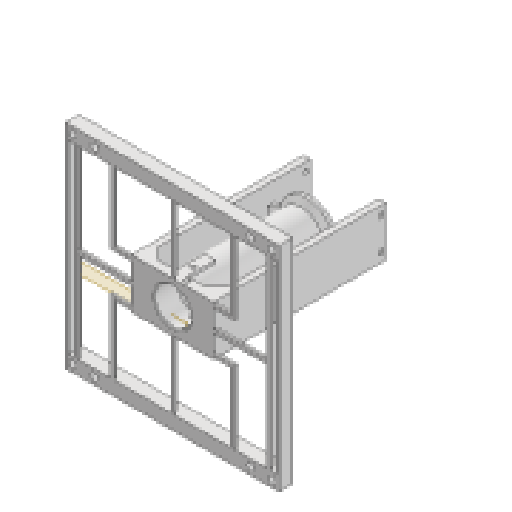
# Autodesk Inventor part: Flexible_tube_bolster_fixed_v3
Saved by Autodesk Inventor 2023 (Build 270158000, 158)
## iProperties
Created: 2021-01-08
Part Number: Flexible_tube_bolster_fixed_v3
Material: Generic
Document SubType Name: Modeling
Designer: CDT
Density: 1 g/cm^3
Appearance: Default
Author: CDT
Autodesk Inventor part; units mm, degrees
ref_plane "YZ Plane" through (0, 0, 0) normal (1, 0, 0) x (0, 1, 0)
ref_plane "XZ Plane" through (0, 0, 0) normal (0, 1, 0) x (-1, 0, 0)
ref_plane "XY Plane" through (0, 0, 0) normal (0, 0, 1) x (1, 0, 0)
ref_plane "Work Plane1" through (0, 0, 0) normal (0, 0, 1) x (1, 0, 0)
sketch "Sketch1" plane through (0, 0, 0) normal (0, 0, 1) x (1, 0, 0)
  line L0 (-30.0874, -48.0547) -> (89.9126, -48.0547)
  line L1 (89.9126, -48.0547) -> (89.9126, 71.9453)
  line L2 (89.9126, 71.9453) -> (-30.0874, 71.9453)
  line L3 (-30.0874, 71.9453) -> (-30.0874, -48.0547)
  circle A0 centre (-26.0874, 67.9453) radius 2
  circle A1 centre (85.9126, 67.9453) radius 2
  circle A2 centre (85.9126, -44.0547) radius 2
  circle A3 centre (-26.0874, -44.0547) radius 2
  circle A4 centre (-14.0874, 67.9453) radius 2
  circle A5 centre (73.9126, 67.9453) radius 2
  circle A6 centre (-14.0874, -44.0547) radius 2
  circle A7 centre (73.9126, -44.0547) radius 2
  point P0 (0, 0)
  dimension "d0" = 120
  dimension "d1" = 120
  dimension "d2" = 4
  dimension "d3" = 4
  dimension "d4" = 4
  dimension "d5" = 4
  dimension "d107" = 4
  dimension "d108" = 4
  dimension "d109" = 4
  dimension "d110" = 4
  dimension "d111" = 4
  dimension "d112" = 4
  dimension "d113" = 4
  dimension "d114" = 4
  dimension "d172" = 4
  dimension "d173" = 4
  dimension "d174" = 4
  dimension "d175" = 4
  dimension "d176" = 16
  dimension "d177" = 4
  dimension "d178" = 4
  dimension "d179" = 16
  dimension "d180" = 16
  dimension "d181" = 4
  dimension "d182" = 4
  dimension "d183" = 16
  constraints: 8 centre point, 8 end point, 2 parallel, 1 horizontal, 1 perpendicular
  measures "d0" distance of L2.end L0.start
  measures "d1" distance of L1.end L2.end
  measures "d2" diameter of A0
  measures "d3" diameter of A1
  measures "d4" diameter of A2
  measures "d5" diameter of A3
  measures "d107" distance from line of L1 A1.centre
  measures "d108" distance from line of L3 A0.centre
  measures "d109" distance from line of L3 A3.centre
  measures "d110" distance from line of L1 A2.centre
  measures "d111" distance from line of L2 A0.centre
  measures "d112" distance from line of L2 A1.centre
  measures "d113" distance from line of L0 A2.centre
  measures "d114" distance from line of L0 A3.centre
  measures "d172" diameter of A4
  measures "d173" diameter of A5
  measures "d174" diameter of A6
  measures "d175" diameter of A7
  measures "d176" distance from line of A6.centre L3
  measures "d177" distance from line of L0 A6.centre
  measures "d178" distance from line of L0 A7.centre
  measures "d179" distance from line of L1 A7.centre
  measures "d180" distance from line of L1 A5.centre
  measures "d181" distance from line of L2 A5.centre
  measures "d182" distance from line of L2 A4.centre
  measures "d183" distance from line of L3 A4.centre
extrude "Extrusion1" add sketch "Sketch1" along normal blind 5
sketch "Sketch2" plane through (0, 0, 5) normal (0, 0, 1) x (1, 0, 0)
  line L0 (-23.0874, -40.0547) -> (6.9126, -40.0547)
  line L1 (6.9126, -40.0547) -> (6.9126, 10.6953)
  line L2 (6.9126, 10.6953) -> (-23.0874, 10.6953)
  line L3 (-23.0874, 10.6953) -> (-23.0874, -40.0547)
  line L4 (89.9126, -48.0547) -> (89.9126, 71.9453) projected
  line L5 (-30.0874, 71.9453) -> (-30.0874, -48.0547) projected
  line L6 (-30.0874, -48.0547) -> (89.9126, -48.0547) projected
  line L7 (89.9126, 71.9453) -> (-30.0874, 71.9453) projected
  line L8 (-23.0874, 13.1953) -> (6.9126, 13.1953)
  line L9 (6.9126, 13.1953) -> (6.9126, 63.9453)
  line L10 (6.9126, 63.9453) -> (-23.0874, 63.9453)
  line L11 (-23.0874, 63.9453) -> (-23.0874, 13.1953)
  line L12 (82.9126, -40.0547) -> (52.9126, -40.0547)
  line L13 (52.9126, -40.0547) -> (52.9126, 10.6953)
  line L14 (52.9126, 10.6953) -> (82.9126, 10.6953)
  line L15 (82.9126, 10.6953) -> (82.9126, -40.0547)
  line L16 (82.9126, 13.1953) -> (52.9126, 13.1953)
  line L17 (52.9126, 13.1953) -> (52.9126, 63.9453)
  line L18 (52.9126, 63.9453) -> (82.9126, 63.9453)
  line L19 (82.9126, 63.9453) -> (82.9126, 13.1953)
  line L20 (-23.0874, -40.0547) -> (82.9126, -40.0547)
  line L21 (82.9126, -40.0547) -> (82.9126, -2.0547)
  line L22 (82.9126, -2.0547) -> (-23.0874, -2.0547)
  line L23 (-23.0874, -2.0547) -> (-23.0874, -40.0547)
  line L24 (-23.0874, 63.9453) -> (82.9126, 63.9453)
  line L25 (82.9126, 63.9453) -> (82.9126, 25.9453)
  line L26 (82.9126, 25.9453) -> (-23.0874, 25.9453)
  line L27 (-23.0874, 25.9453) -> (-23.0874, 63.9453)
  line L28 (82.9126, 11.9453) -> (52.9126, 11.9453)
  line L29 (52.9126, 11.9453) -> (52.9126, 11.9453)
  line L30 (52.9126, 11.9453) -> (82.9126, 11.9453)
  line L31 (82.9126, 11.9453) -> (82.9126, 11.9453)
  line L32 (11.9126, 11.9453) -> (-23.0874, 11.9453)
  line L33 (-23.0874, 11.9453) -> (-23.0874, 11.9453)
  line L34 (-23.0874, 11.9453) -> (11.9126, 11.9453)
  line L35 (11.9126, 11.9453) -> (11.9126, 11.9453)
  line L36 (-25.5874, -40.0547) -> (-30.0874, -40.0547)
  line L37 (-30.0874, -40.0547) -> (-30.0874, 63.9453)
  line L38 (-30.0874, 63.9453) -> (-25.5874, 63.9453)
  line L39 (-25.5874, 63.9453) -> (-25.5874, -40.0547)
  line L40 (89.9126, 63.9453) -> (85.4126, 63.9453)
  line L41 (85.4126, 63.9453) -> (85.4126, -40.0547)
  line L42 (85.4126, -40.0547) -> (89.9126, -40.0547)
  line L43 (89.9126, -40.0547) -> (89.9126, 63.9453)
  line L44 (-30.0874, -48.0547) -> (-44.0088, -48.0547)
  line L45 (-44.0088, -48.0547) -> (-44.0088, 71.9453)
  line L46 (-44.0088, 71.9453) -> (-30.0874, 71.9453)
  line L47 (-30.0874, 71.9453) -> (-30.0874, -48.0547)
  point P0 (0, 0)
  point P1 (6.9126, 63.9453)
  point P2 (6.9126, 25.9453)
  point P3 (52.9126, 25.9453)
  point P4 (52.9126, -2.0547)
  point P5 (6.9126, -2.0547)
  point P6 (-30.0874, 63.9453)
  point P7 (-30.0874, -40.0547)
  point P8 (89.9126, -40.0547)
  dimension "d9" = 7
  dimension "d10" = 8
  dimension "d13" = 8
  dimension "d15" = 7
  dimension "d19" = 7
  dimension "d20" = 7
  dimension "d21" = 8
  dimension "d23" = 7
  dimension "d24" = 58.75
  dimension "d25" = 58.75
  dimension "d26" = 38
  dimension "d27" = 38
  dimension "d28" = 30
  dimension "d29" = 30
  dimension "d30" = 30
  dimension "d31" = 58.75
  dimension "d32" = 58.75
  dimension "d33" = 30
  dimension "d54" = 1.25
  dimension "d55" = 1.25
  dimension "d56" = 7
  dimension "d57" = 35
  dimension "d58" = 7
  dimension "d91" = 0
  dimension "d115" = 8
  dimension "d116" = 8
  dimension "d117" = 2.5
  dimension "d119" = 8
  dimension "d120" = 8
  dimension "d121" = 2.5
  dimension "d168" = 28
  dimension "d342" = 120
  dimension "d352" = 120
  dimension "d775" = 46
  constraints: 88 end point, 22 equal length, 11 horizontal, 11 perpendicular, 5 point on line, 3 collinear
  measures "d9" distance between parallel lines of L5 L3
  measures "d10" distance between parallel lines of L6 L0
  measures "d13" distance between parallel lines of L7 L10
  measures "d15" distance between parallel lines of L5 L11
  measures "d19" distance between parallel lines of L21 L4
  measures "d20" distance between parallel lines of L4 L15
  measures "d21" distance between parallel lines of L6 L12
  measures "d23" distance between parallel lines of L4 L19
  measures "d24" distance between parallel lines of L6 L14
  measures "d25" distance between parallel lines of L16 L7
  measures "d26" distance between parallel lines of L26 L24
  measures "d27" distance between parallel lines of L22 L20
  measures "d28" distance between parallel lines of L13 L15
  measures "d29" distance between parallel lines of L17 L19
  measures "d30" distance between parallel lines of L1 L3
  measures "d31" distance between parallel lines of L6 L2
  measures "d32" distance between parallel lines of L8 L7
  measures "d33" distance between parallel lines of L9 L11
  measures "d54" distance between parallel lines of L14 L28
  measures "d55" distance between parallel lines of L16 L30
  measures "d56" distance between parallel lines of L4 L31
  measures "d57" distance between parallel lines of L33 L35
  measures "d58" distance between parallel lines of L5 L33
  measures "d91" distance between parallel lines of L32 L34
  measures "d115" distance between parallel lines of L6 L36
  measures "d116" distance between parallel lines of L7 L38
  measures "d117" distance between parallel lines of L11 L39
  measures "d119" distance between parallel lines of L7 L40
  measures "d120" distance between parallel lines of L6 L42
  measures "d121" distance between parallel lines of L19 L41
  measures "d168" distance between parallel lines of L26 L22
  measures "d342" distance of L4.end L5.start
  measures "d352" distance of L44.end L45.end
  measures "d775" distance between parallel lines of L13 L1
extrude "Extrusion2" cut sketch "Sketch2" against normal blind 10 contours L3 L22 L1 L0 | L1 L22 L13 L20 | L3 L2 L1 L22 | L13 L22 L15 L12 | L13 L14 L15 L22 | L42 L41 L40 L4 | L5 L38 L39 L36 | L11 L26 L9 L8 | L11 L10 L9 L26 | L9 L24 L17 L26 | L26 L19 L16 L17 | L17 L18 L19 L26
sketch "Sketch4" plane through (89.9126, -48.0547, 0) normal (1, 0, 0) x (0, 0, -1)
  line L0 (0, 8) -> (-3.6, 8)
  line L1 (-3.6, 8) -> (-3.6, 76)
  line L2 (-3.6, 76) -> (0, 76)
  line L3 (0, 76) -> (0, 8)
  line L4 (0, 0) -> (0, 120) projected
  line L5 (0, 112) -> (-3.6, 112)
  line L6 (-3.6, 112) -> (-3.6, 44)
  line L7 (-3.6, 44) -> (0, 44)
  line L8 (0, 44) -> (0, 112)
  line L9 (0, 120) -> (-5, 120) projected
  line L10 (-5, 0) -> (-5, 120) projected
  point P0 (0, 44)
  dimension "d49" = 68
  dimension "d51" = 68
  dimension "d59" = 8
  dimension "d71" = 1.4
  dimension "d72" = 1.4
  constraints: 16 end point, 4 parallel, 2 horizontal, 2 perpendicular, 1 point on line
  measures "d49" distance of L0.end L1.end
  measures "d51" distance of L6.end L5.end
  measures "d59" distance between parallel lines of L9 L5
  measures "d71" distance between parallel lines of L10 L6
  measures "d72" distance between parallel lines of L10 L1
extrude "Extrusion4" cut sketch "Sketch4" against normal up to surface (37 mm away)
sketch "Sketch5" plane through (-30.0874, -48.0547, 0) normal (-1, 0, 0) x (0, 0, 1)
  line L0 (3.0594, 112) -> (0.0594, 112)
  line L1 (0, 112) -> (3.6, 112)
  line L2 (3.6, 112) -> (3.6, 44)
  line L3 (3.6, 44) -> (0, 44)
  line L4 (0, 44) -> (0, 112)
  line L5 (0, 8) -> (3.6, 8)
  line L6 (3.6, 8) -> (3.6, 76)
  line L7 (3.6, 76) -> (0, 76)
  line L8 (0, 76) -> (0, 8)
  line L9 (0, 120) -> (5, 120) projected
  line L10 (0, 120) -> (0, 0) projected
  line L11 (5, 120) -> (5, 0) projected
  point P0 (0, 48.0547)
  point P1 (2.7, 132)
  point P2 (3.6, 76)
  dimension "d62" = 68
  dimension "d66" = 68
  dimension "d68" = 8
  dimension "d69" = 1.4
  dimension "d70" = 1.4
  constraints: 18 end point, 4 parallel, 2 horizontal, 2 perpendicular, 1 collinear, 1 point on line
  measures "d62" distance of L1.end L2.end
  measures "d66" distance of L6.end L5.end
  measures "d68" distance between parallel lines of L9 L0
  measures "d69" distance between parallel lines of L11 L2
  measures "d70" distance between parallel lines of L11 L6
extrude "Extrusion5" cut sketch "Sketch5" against normal up to surface (37 mm away)
sketch "Sketch34" plane through (0, 0, 5) normal (0, 0, 1) x (1, 0, 0)
  line L0 (-5.0874, 63.9453) -> (-3.0874, 63.9453)
  line L1 (-3.0874, 63.9453) -> (-3.0874, 22.9453)
  line L2 (-3.0874, 22.9453) -> (-5.0874, 22.9453)
  line L3 (-5.0874, 22.9453) -> (-5.0874, 63.9453)
  line L4 (-23.0874, 63.9453) -> (82.9126, 63.9453) projected
  line L5 (-23.0874, 13.1953) -> (-23.0874, 63.9453) projected
  line L6 (62.9126, 63.9453) -> (64.9126, 63.9453)
  line L7 (64.9126, 63.9453) -> (64.9126, 22.9453)
  line L8 (64.9126, 22.9453) -> (62.9126, 22.9453)
  line L9 (62.9126, 22.9453) -> (62.9126, 63.9453)
  line L10 (82.9126, 63.9453) -> (82.9126, 13.1953) projected
  line L11 (-3.0874, 22.9453) -> (6.9126, 22.9453)
  line L12 (6.9126, 22.9453) -> (6.9126, 24.9453)
  line L13 (6.9126, 24.9453) -> (-3.0874, 24.9453)
  line L14 (-3.0874, 24.9453) -> (-3.0874, 22.9453)
  line L15 (62.9126, 22.9453) -> (52.9126, 22.9453)
  line L16 (52.9126, 22.9453) -> (52.9126, 24.9453)
  line L17 (52.9126, 24.9453) -> (62.9126, 24.9453)
  line L18 (62.9126, 24.9453) -> (62.9126, 22.9453)
  line L19 (-5.0874, -40.0547) -> (-3.0874, -40.0547)
  line L20 (-3.0874, -40.0547) -> (-3.0874, 0.9453)
  line L21 (-3.0874, 0.9453) -> (-5.0874, 0.9453)
  line L22 (-5.0874, 0.9453) -> (-5.0874, -40.0547)
  line L23 (62.9126, -40.0547) -> (64.9126, -40.0547)
  line L24 (64.9126, -40.0547) -> (64.9126, 0.9453)
  line L25 (64.9126, 0.9453) -> (62.9126, 0.9453)
  line L26 (62.9126, 0.9453) -> (62.9126, -40.0547)
  line L27 (-23.0874, -40.0547) -> (-23.0874, 10.6953) projected
  line L28 (-3.0874, 0.9453) -> (6.9126, 0.9453)
  line L29 (6.9126, 0.9453) -> (6.9126, -1.0547)
  line L30 (6.9126, -1.0547) -> (-3.0874, -1.0547)
  line L31 (-3.0874, -1.0547) -> (-3.0874, 0.9453)
  line L32 (82.9126, 10.6953) -> (82.9126, -40.0547) projected
  line L33 (62.9126, 0.9453) -> (52.9126, 0.9453)
  line L34 (52.9126, 0.9453) -> (52.9126, -1.0547)
  line L35 (52.9126, -1.0547) -> (62.9126, -1.0547)
  line L36 (62.9126, -1.0547) -> (62.9126, 0.9453)
  line L37 (-30.0874, -48.0547) -> (89.9126, -48.0547) projected
  line L38 (89.9126, -48.0547) -> (-30.0874, -48.0547)
  line L39 (-30.0874, -48.0547) -> (-30.0874, -57.7562)
  line L40 (-30.0874, -57.7562) -> (89.9126, -57.7562)
  line L41 (89.9126, -57.7562) -> (89.9126, -48.0547)
  line L42 (-30.0874, 71.9453) -> (-30.0874, -48.0547) projected
  line L43 (-30.0874, -48.0547) -> (-47.0069, -48.0547)
  line L44 (-47.0069, -48.0547) -> (-47.0069, 71.9453)
  line L45 (-47.0069, 71.9453) -> (-30.0874, 71.9453)
  line L46 (-30.0874, 71.9453) -> (-30.0874, -48.0547)
  line L47 (-30.0874, 71.9453) -> (-30.0874, -48.0547) projected
  line L48 (89.9126, 71.9453) -> (-30.0874, 71.9453) projected
  line L49 (-23.0874, -40.0547) -> (82.9126, -40.0547) projected
  line L50 (52.9126, -2.0547) -> (52.9126, 10.6953) projected
  line L51 (52.9126, -2.0547) -> (52.9126, 10.6953) projected
  line L52 (6.9126, 10.6953) -> (6.9126, -2.0547) projected
  line L53 (6.9126, 10.6953) -> (6.9126, -2.0547) projected
  point P0 (-3.0874, 24.9453)
  point P1 (-3.0874, -1.0547)
  point P2 (-30.0874, -40.0547)
  point P3 (89.9126, -40.0547)
  point P4 (52.9126, 13.1953)
  point P5 (52.9126, 25.9453)
  point P6 (6.9126, 25.9453)
  point P7 (6.9126, 13.1953)
  dimension "d317" = 0
  dimension "d318" = 41
  dimension "d319" = 18
  dimension "d320" = 2
  dimension "d321" = 2
  dimension "d322" = 41
  dimension "d323" = 0
  dimension "d324" = 18
  dimension "d326" = 2
  dimension "d328" = 2
  dimension "d329" = 18
  dimension "d330" = 2
  dimension "d333" = 2
  dimension "d335" = 18
  dimension "d336" = 2
  dimension "d337" = 41
  dimension "d339" = 2
  dimension "d364" = 120
  dimension "d365" = 120
  dimension "d373" = 41
  dimension "d374" = 41
  constraints: 80 end point, 20 parallel, 10 horizontal, 10 perpendicular, 6 collinear
  measures "d317" distance between parallel lines of L4 L0
  measures "d318" distance between parallel lines of L2 L0
  measures "d319" distance between parallel lines of L3 L5
  measures "d320" distance between parallel lines of L1 L3
  measures "d321" distance of L7.end L8.end
  measures "d322" distance of L6.end L7.end
  measures "d323" distance between parallel lines of L4 L6
  measures "d324" distance between parallel lines of L10 L7
  measures "d326" distance of L12.end L11.end
  measures "d328" distance of L15.end L16.end
  measures "d329" distance between parallel lines of L27 L22
  measures "d330" distance between parallel lines of L20 L22
  measures "d333" distance of L28.end L29.end
  measures "d335" distance between parallel lines of L32 L24
  measures "d336" distance between parallel lines of L26 L24
  measures "d337" distance between parallel lines of L25 L23
  measures "d339" distance of L34.end L33.end
  measures "d364" distance of L42.start L37.start
  measures "d365" distance of L39.end L40.end
  measures "d373" distance between parallel lines of L49 L28
  measures "d374" distance between parallel lines of L49 L33
extrude "Extrusion32" add sketch "Sketch34" against normal blind 1.4 contours L0 L1 L2 L3 | L13 L12 L11 L1 | L4 L7 L8 L9 | L9 L15 L16 L17 | L22 L21 L20 L19 | L20 L28 L29 L30 | L26 L25 L24 L23 | L35 L34 L33 L26
sketch "Sketch48" plane through (0, 0, 0) normal (0, 0, -1) x (-1, 0, 0)
  circle A0 centre (-29.9126, 11.9453) radius 10.2
  line L0 (-52.9126, -2.0547) -> (-6.9126, -2.0547) projected
  line L1 (-6.9126, 25.9453) -> (-52.9126, 25.9453) projected
  line L2 (-52.9126, 10.6953) -> (-52.9126, -2.0547) projected
  line L3 (-6.9126, -2.0547) -> (-6.9126, 10.6953) projected
  line L4 (-89.9126, 71.9453) -> (30.0874, 71.9453) projected
  line L5 (30.0874, -48.0547) -> (-89.9126, -48.0547) projected
  line L6 (-52.9126, 25.9453) -> (-6.9126, 25.9453) projected
  line L7 (-52.9126, -2.0547) -> (-6.9126, -2.0547)
  line L8 (-6.9126, -2.0547) -> (-6.9126, 25.9453)
  line L9 (-6.9126, 25.9453) -> (-52.9126, 25.9453)
  line L10 (-52.9126, 25.9453) -> (-52.9126, -2.0547)
  point P0 (0, 0)
  point P1 (-16.9126, 41.9453)
  point P2 (-52.9126, 41.9453)
  point P3 (-6.9126, 10.6953)
  dimension "d489" = 20.4
  dimension "d542" = 60
  dimension "d543" = 60
  dimension "d544" = 14
  dimension "d545" = 28
  dimension "d546" = 46
  dimension "d547" = 23
  constraints: 8 end point, 2 parallel, 1 centre point, 1 horizontal, 1 perpendicular, 2 other
  measures "d489" diameter of A0
  measures "d542" distance from line of L4 A0.centre
  measures "d543" distance from line of L5 A0.centre
  measures "d545" distance of L9.end L0.start
  measures "d546" distance of L6.end L6.start
  measures "d547" distance from line of L8 A0.centre
extrude "Extrusion46" cut sketch "Sketch48" against normal blind 10 contours A0
sketch "Sketch52" plane through (0, 0, 5) normal (0, 0, 1) x (1, 0, 0)
  line L0 (28.9126, 25.9453) -> (30.9126, 25.9453)
  line L1 (30.9126, 25.9453) -> (30.9126, 63.9453)
  line L2 (30.9126, 63.9453) -> (28.9126, 63.9453)
  line L3 (28.9126, 63.9453) -> (28.9126, 25.9453)
  line L4 (28.9126, -2.0547) -> (30.9126, -2.0547)
  line L5 (30.9126, -2.0547) -> (30.9126, -40.0547)
  line L6 (30.9126, -40.0547) -> (28.9126, -40.0547)
  line L7 (28.9126, -40.0547) -> (28.9126, -2.0547)
  line L8 (-30.0874, 71.9453) -> (-30.0874, -48.0547) projected
  line L9 (89.9126, -48.0547) -> (89.9126, 71.9453) projected
  line L10 (82.9126, -40.0547) -> (-23.0874, -40.0547) projected
  line L11 (6.9126, -2.0547) -> (52.9126, -2.0547) projected
  line L12 (-23.0874, 63.9453) -> (82.9126, 63.9453) projected
  line L13 (52.9126, 25.9453) -> (6.9126, 25.9453) projected
  line L14 (-30.0874, 71.9453) -> (-30.0874, -48.0547) projected
  line L15 (89.9126, -48.0547) -> (89.9126, 71.9453) projected
  line L16 (-30.0874, -48.0547) -> (89.9126, -48.0547) projected
  line L17 (89.9126, -48.0547) -> (-30.0874, -48.0547)
  line L18 (-30.0874, -48.0547) -> (-30.0874, -57.7826)
  line L19 (-30.0874, -57.7826) -> (89.9126, -57.7826)
  line L20 (89.9126, -57.7826) -> (89.9126, -48.0547)
  point P0 (0, 0)
  point P1 (-30.0874, -40.0547)
  point P2 (99.9126, -40.0547)
  point P3 (62.9126, -40.0547)
  point P4 (-3.0874, -40.0547)
  point P5 (-3.0874, 63.9453)
  point P6 (62.9126, 63.9453)
  point P7 (52.9126, 41.9453)
  point P8 (16.9126, 41.9453)
  point P9 (-30.0874, 73.9453)
  point P10 (99.9126, 73.9453)
  point P11 (89.9126, 71.9453)
  point P12 (-25.3874, -40.0547)
  point P13 (95.2126, 73.9453)
  point P14 (6.9126, 25.9453)
  point P15 (6.9126, 25.9453)
  dimension "d520" = 59
  dimension "d521" = 59
  dimension "d522" = 0
  dimension "d523" = 0
  dimension "d524" = 0
  dimension "d525" = 0
  dimension "d526" = 59
  dimension "d527" = 59
  dimension "d636" = 2
  dimension "d776" = 120
  constraints: 24 end point, 6 parallel, 3 horizontal, 3 perpendicular, 4 other
  measures "d520" distance between parallel lines of L7 L8
  measures "d522" distance between parallel lines of L10 L6
  measures "d523" distance between parallel lines of L11 L4
  measures "d524" vertical extent of L2
  measures "d525" vertical extent of L0
  measures "d526" distance between parallel lines of L14 L3
  measures "d636" distance between parallel lines of L3 L1
  measures "d776" distance of L18.end L19.end
extrude "Extrusion50" add sketch "Sketch52" against normal blind 1.25 contours L3 L2 L1 L0 | L4 L5 L6 L7
sketch "Sketch57" plane through (0, 0, 0) normal (0, 0, -1) x (-1, 0, 0)
  circle A0 centre (-29.9126, 11.9453) radius 10.2 projected
  circle A1 centre (-29.9126, 11.9453) radius 10
  circle A2 centre (-29.9126, 11.9453) radius 12.5
  point P0 (0, 0)
  dimension "d576" = 25
  dimension "d601" = 20
  constraints: 2 centre point, 2 coincident
  measures "d576" diameter of A2
  measures "d601" diameter of A1
extrude "Extrusion55" add sketch "Sketch57" along normal blind 72.4 contours A2
sketch "Sketch58" plane through (0, 0, 0) normal (0, 0, -1) x (-1, 0, 0)
  line L0 (-10.5126, 25.9453) -> (-6.9126, 25.9453)
  line L1 (-6.9126, 25.9453) -> (-6.9126, -2.0547)
  line L2 (-6.9126, -2.0547) -> (-10.5126, -2.0547)
  line L3 (-10.5126, -2.0547) -> (-10.5126, 25.9453)
  line L4 (-52.9126, -2.0547) -> (-6.9126, -2.0547) projected
  line L5 (-6.9126, 25.9453) -> (-52.9126, 25.9453) projected
  line L6 (-6.9126, -2.0547) -> (-6.9126, 10.6953) projected
  line L7 (-52.9126, 25.9453) -> (-49.3126, 25.9453)
  line L8 (-49.3126, 25.9453) -> (-49.3126, -2.0547)
  line L9 (-49.3126, -2.0547) -> (-52.9126, -2.0547)
  line L10 (-52.9126, -2.0547) -> (-52.9126, 25.9453)
  line L11 (-52.9126, 10.6953) -> (-52.9126, -2.0547) projected
  point P0 (0, 0)
  point P1 (-11.9126, 30.9453)
  point P2 (-6.9126, 10.6953)
  dimension "d579" = 0
  dimension "d582" = 3.6
  dimension "d583" = 0
  dimension "d586" = 3.6
  constraints: 16 end point, 4 parallel, 2 horizontal, 2 perpendicular, 2 other
  measures "d579" distance between parallel lines of L4 L2
  measures "d582" distance between parallel lines of L1 L3
  measures "d583" distance between parallel lines of L4 L9
  measures "d586" distance between parallel lines of L8 L10
extrude "Extrusion56" add sketch "Sketch58" along normal blind 91.8 contours L0 L1 L2 L3 | L8 L4 L10 L5
sketch "Sketch59" plane through (52.9126, -2.0547, 5) normal (1, 0, 0) x (0, 0, -1)
  circle A0 centre (94.3, 5) radius 1.55
  circle A1 centre (94.3, 23) radius 1.55
  line L0 (0, 0) -> (96.8, 0) projected
  line L1 (96.8, 28) -> (96.8, 0) projected
  line L2 (0, 28) -> (96.8, 28) projected
  point P0 (5, 2.0547)
  point P1 (5, 1)
  point P2 (5, 27)
  dimension "d589" = 3.1
  dimension "d590" = 3.1
  dimension "d591" = 18
  dimension "d592" = 5
  dimension "d593" = 2.5
  dimension "d594" = 2.5
  dimension "d595" = 5
  constraints: 2 centre point, 2 other
  measures "d589" diameter of A0
  measures "d590" diameter of A1
  measures "d591" distance of A0.centre A1.centre
  measures "d593" distance from line of L1 A0.centre
  measures "d594" distance from line of L1 A1.centre
extrude "Extrusion57" cut sketch "Sketch59" against normal through all
sketch "Sketch61" plane through (0, 0, 0) normal (0, 0, -1) x (-1, 0, 0)
  line L0 (30.0874, -48.0547) -> (-89.9126, -48.0547) projected
  line L1 (23.0874, -40.0547) -> (-82.9126, -40.0547) projected
  line L2 (-89.9126, -48.0547) -> (30.0874, -48.0547)
  line L3 (30.0874, -48.0547) -> (30.0874, -40.0547)
  line L4 (30.0874, -40.0547) -> (-89.9126, -40.0547)
  line L5 (-89.9126, -40.0547) -> (-89.9126, -48.0547)
  circle A0 centre (-85.9126, 67.9453) radius 2 projected
  circle A1 centre (-85.9126, 67.9453) radius 2
  circle A2 centre (-73.9126, 67.9453) radius 2 projected
  circle A3 centre (-73.9126, 67.9453) radius 2
  circle A4 centre (14.0874, 67.9453) radius 2 projected
  circle A5 centre (14.0874, 67.9453) radius 2
  circle A6 centre (26.0874, 67.9453) radius 2 projected
  circle A7 centre (26.0874, 67.9453) radius 2
  circle A8 centre (26.0874, -44.0547) radius 2 projected
  circle A9 centre (26.0874, -44.0547) radius 2
  circle A10 centre (14.0874, -44.0547) radius 2 projected
  circle A11 centre (14.0874, -44.0547) radius 2
  circle A12 centre (-73.9126, -44.0547) radius 2 projected
  circle A13 centre (-73.9126, -44.0547) radius 2
  circle A14 centre (-85.9126, -44.0547) radius 2 projected
  circle A15 centre (-85.9126, -44.0547) radius 2
  line L6 (23.0874, 63.9453) -> (-82.9126, 63.9453) projected
  line L7 (-89.9126, 71.9453) -> (30.0874, 71.9453) projected
  line L8 (-89.9126, 63.9453) -> (30.0874, 63.9453)
  line L9 (30.0874, 63.9453) -> (30.0874, 71.9453)
  line L10 (30.0874, 71.9453) -> (-89.9126, 71.9453)
  line L11 (-89.9126, 71.9453) -> (-89.9126, 63.9453)
  point P0 (0, 0)
  point P1 (-99.9126, -40.0547)
  point P2 (-99.9126, -40.0547)
  point P3 (30.0874, -48.0547)
  point P4 (-85.4126, 63.9453)
  point P5 (-85.4126, 63.9453)
  constraints: 16 end point, 8 centre point, 8 coincident, 4 parallel, 2 horizontal, 2 perpendicular
extrude "Extrusion59" add sketch "Sketch61" along normal blind 2.5
sketch "Sketch62" plane through (0, 0, 5) normal (0, 0, 1) x (1, 0, 0)
  circle A0 centre (29.9126, 11.9453) radius 10.2 projected
  circle A1 centre (29.9126, 11.9453) radius 10.2
  circle A2 centre (29.9126, 11.9453) radius 7.75
  point P0 (0, 0)
  dimension "d609" = 15.5
  constraints: 2 centre point, 2 coincident
  measures "d609" diameter of A2
extrude "Extrusion60" add sketch "Sketch62" against normal blind 18
sketch "Sketch63" plane through (0, 0, 5) normal (0, 0, 1) x (1, 0, 0)
  circle A0 centre (29.9126, 11.9453) radius 7.75 projected
  circle A1 centre (29.9126, 11.9453) radius 10.275
  point P0 (0, 0)
  dimension "d612" = 20.55
  constraints: 1 centre point, 1 coincident
  measures "d612" diameter of A1
extrude "Extrusion61" cut sketch "Sketch63" against normal blind 13
sketch "Sketch64" plane through (29.9126, 11.9453, -72.4) normal (0, 0, -1) x (-1, 0, 0)
  line L0 (-10.4, 3) -> (-19.4, 3)
  line L1 (-19.4, 3) -> (-19.4, -3)
  line L2 (-19.4, -3) -> (-10.4, -3)
  line L3 (-10.4, -3) -> (-10.4, 3)
  line L4 (19.4, 3) -> (10.4, 3)
  line L5 (10.4, 3) -> (10.4, -3)
  line L6 (10.4, -3) -> (19.4, -3)
  line L7 (19.4, -3) -> (19.4, 3)
  line L8 (19.4, 14) -> (-19.4, 14) projected
  line L9 (-23, -14) -> (23, -14) projected
  line L10 (19.4, 14) -> (19.4, -14) projected
  line L11 (-19.4, -14) -> (-19.4, 14) projected
  point P0 (29.9126, -11.9453)
  point P1 (23, 14)
  point P2 (-23, 14)
  point P3 (19.4, 14)
  point P4 (19.4, -14)
  point P5 (-19.4, -14)
  point P6 (-19.4, 14)
  point P7 (10.4, 14)
  point P8 (-10.4, 14)
  dimension "d618" = 11
  dimension "d619" = 11
  dimension "d620" = 11
  dimension "d621" = 0
  dimension "d622" = 9
  dimension "d623" = 9
  dimension "d624" = 0
  constraints: 16 end point, 4 parallel, 2 horizontal, 2 perpendicular, 1 point on line
  measures "d618" distance between parallel lines of L8 L4
  measures "d619" distance between parallel lines of L9 L6
  measures "d620" distance between parallel lines of L9 L2
  measures "d621" distance between parallel lines of L10 L7
  measures "d622" distance between parallel lines of L5 L7
  measures "d623" distance between parallel lines of L11 L3
  measures "d624" distance between parallel lines of L11 L1
extrude "Extrusion62" add sketch "Sketch64" against normal blind 1 contours L3 L2 L1 L0 | L7 L6 L5 L4
chamfer "Chamfer11" distance 3.5 angle 45 5 edges at (42.4126, 11.9453, -71.4) (49.3126, 11.9453, -71.4) (17.5042, 10.4342, -71.4) (17.5042, 13.4564, -71.4) (10.5126, 11.9453, -71.4)
sketch "Sketch65" plane through (0, 0, -72.4) normal (0, 0, -1) x (-1, 0, 0)
  circle A0 centre (-29.9126, 11.9453) radius 10.2 projected
  circle A1 centre (-29.9126, 11.9453) radius 10.2
  circle A2 centre (-29.9126, 11.9453) radius 15.5
  point P0 (0, 0)
  dimension "d630" = 31
  constraints: 2 centre point, 2 coincident
  measures "d630" diameter of A2
extrude "Extrusion63" add sketch "Sketch65" against normal blind 2
chamfer "Chamfer12" distance 3 angle 45 2 edges at (29.9126, 24.4453, -70.4) (29.9126, -0.5547, -70.4)
chamfer "Chamfer20" distance 6 angle 45 2 edges at (10.5126, 11.9453, 0) (49.3126, 11.9453, 0)
sketch "Sketch71" plane through (0, 0, 0) normal (0, 0, -1) x (-1, 0, 0)
  line L0 (-26.9126, -2.0547) -> (-32.9126, -2.0547)
  line L1 (-32.9126, -2.0547) -> (-32.9126, 0.1453)
  line L2 (-32.9126, 0.1453) -> (-26.9126, 0.1453)
  line L3 (-26.9126, 0.1453) -> (-26.9126, -2.0547)
  line L4 (-52.9126, -2.0547) -> (-6.9126, -2.0547) projected
  line L5 (-6.9126, 10.6953) -> (-6.9126, -2.0547) projected
  line L6 (-52.9126, -2.0547) -> (-52.9126, 10.6953) projected
  line L7 (-26.9126, 25.9453) -> (-32.9126, 25.9453)
  line L8 (-32.9126, 25.9453) -> (-32.9126, 23.7453)
  line L9 (-32.9126, 23.7453) -> (-26.9126, 23.7453)
  line L10 (-26.9126, 23.7453) -> (-26.9126, 25.9453)
  line L11 (-6.9126, 10.6953) -> (-6.9126, -2.0547) projected
  line L12 (-6.9126, 25.9453) -> (-52.9126, 25.9453) projected
  line L13 (-52.9126, -2.0547) -> (-52.9126, 10.6953) projected
  point P0 (0, 0)
  point P1 (-43.3126, -2.0547)
  point P2 (-16.5126, -2.0547)
  point P3 (-6.9126, 0.9453)
  point P4 (-52.9126, 0.9453)
  point P5 (-6.9126, 24.9453)
  point P6 (-16.5126, 25.9453)
  point P7 (-43.3126, 25.9453)
  point P8 (-52.9126, 24.9453)
  point P9 (-49.3126, -2.0547)
  point P10 (-10.5126, -2.0547)
  point P11 (-10.5126, 25.9453)
  point P12 (-49.3126, 25.9453)
  dimension "d690" = 0
  dimension "d691" = 2.2
  dimension "d692" = 20
  dimension "d693" = 20
  dimension "d739" = 20
  dimension "d740" = 0
  dimension "d741" = 20
  dimension "d742" = 2.2
  constraints: 16 end point, 4 parallel, 2 horizontal, 2 perpendicular
  measures "d690" distance between parallel lines of L4 L0
  measures "d691" distance between parallel lines of L2 L0
  measures "d692" distance between parallel lines of L3 L5
  measures "d693" distance between parallel lines of L6 L1
  measures "d739" distance between parallel lines of L11 L10
  measures "d740" distance between parallel lines of L12 L7
  measures "d741" distance between parallel lines of L8 L13
  measures "d742" distance between parallel lines of L9 L7
extrude "Extrusion69" add sketch "Sketch71" along normal blind 16
sketch "Sketch72" plane through (6.9126, -2.0547, 5) normal (0, -1, 0) x (1, 0, 0)
  circle A0 centre (23, -11.4) radius 1.5
  line L0 (26, -21) -> (20, -21) projected
  line L1 (26, -5) -> (26, -21) projected
  line L2 (20, -5) -> (20, -21) projected
  line L3 (0, 0) -> (46, 0) projected
  circle A1 centre (23, -4.25) radius 1.5
  line L4 (24, -1.25) -> (22, -1.25) projected
  circle A2 centre (28, -3) radius 1.5
  line L5 (24, 0) -> (24, -1.25) projected
  point P0 (-6.9126, -5)
  point P1 (22, 0)
  point P2 (27.25, -1.25)
  point P3 (18.75, -1.25)
  dimension "d696" = 3
  dimension "d698" = 3
  dimension "d699" = 3
  dimension "d735" = 11.4
  dimension "d736" = 3
  dimension "d738" = 3
  dimension "d759" = 3
  dimension "d791" = 3
  dimension "d792" = 4
  dimension "d793" = 3
  constraints: 3 centre point
  measures "d696" diameter of A0
  measures "d698" distance from line of L1 A0.centre
  measures "d699" distance from line of L2 A0.centre
  measures "d735" distance from line of L3 A0.centre
  measures "d736" diameter of A1
  measures "d738" distance from line of L1 A1.centre
  measures "d759" distance from line of L4 A1.centre
  measures "d791" distance from line of L3 A2.centre
  measures "d792" distance from line of L5 A2.centre
  measures "d793" diameter of A2
extrude "Extrusion70" cut sketch "Sketch72" against normal up to surface (28 mm away) contours A0 | A2
sketch "Sketch73" plane through (0, 0, 5) normal (0, 0, 1) x (1, 0, 0)
  line L0 (85.4126, -40.0547) -> (-25.5874, -40.0547)
  line L1 (-25.5874, -40.0547) -> (-25.5874, -39.0547)
  line L2 (-25.5874, -39.0547) -> (85.4126, -39.0547)
  line L3 (85.4126, -39.0547) -> (85.4126, -40.0547)
  line L4 (85.4126, -40.0547) -> (85.4126, 63.9453) projected
  line L5 (82.9126, -40.0547) -> (-23.0874, -40.0547) projected
  line L6 (-25.5874, 63.9453) -> (-25.5874, -40.0547) projected
  line L7 (85.4126, 63.9453) -> (-25.5874, 63.9453)
  line L8 (-25.5874, 63.9453) -> (-25.5874, 62.9453)
  line L9 (-25.5874, 62.9453) -> (85.4126, 62.9453)
  line L10 (85.4126, 62.9453) -> (85.4126, 63.9453)
  line L11 (-23.0874, 63.9453) -> (82.9126, 63.9453) projected
  line L12 (53.9126, -1.0547) -> (52.9126, -1.0547)
  line L13 (52.9126, -1.0547) -> (52.9126, 24.9453)
  line L14 (52.9126, 24.9453) -> (53.9126, 24.9453)
  line L15 (53.9126, 24.9453) -> (53.9126, -1.0547)
  line L16 (5.9126, -1.0547) -> (6.9126, -1.0547)
  line L17 (6.9126, -1.0547) -> (6.9126, 24.9453)
  line L18 (6.9126, 24.9453) -> (5.9126, 24.9453)
  line L19 (5.9126, 24.9453) -> (5.9126, -1.0547)
  line L20 (52.9126, -2.0547) -> (52.9126, 10.6953) projected
  line L21 (52.9126, -1.0547) -> (62.9126, -1.0547) projected
  line L22 (62.9126, 24.9453) -> (52.9126, 24.9453) projected
  line L23 (6.9126, 24.9453) -> (-3.0874, 24.9453) projected
  line L24 (6.9126, 10.6953) -> (6.9126, -2.0547) projected
  line L25 (-3.0874, -1.0547) -> (6.9126, -1.0547) projected
  line L26 (28.4126, 25.9453) -> (31.4126, 25.9453) projected
  line L27 (30.9126, 25.9453) -> (28.9126, 25.9453)
  line L28 (28.9126, 25.9453) -> (28.9126, 26.9453)
  line L29 (28.9126, 26.9453) -> (30.9126, 26.9453)
  line L30 (30.9126, 26.9453) -> (30.9126, 25.9453)
  line L31 (30.9126, -2.0547) -> (30.9126, -40.0547) projected
  line L32 (30.9126, -2.0547) -> (28.9126, -2.0547)
  line L33 (28.9126, -2.0547) -> (28.9126, -3.0547)
  line L34 (28.9126, -3.0547) -> (30.9126, -3.0547)
  line L35 (30.9126, -3.0547) -> (30.9126, -2.0547)
  point P0 (0, 0)
  point P1 (64.9126, -40.0547)
  point P2 (-25.3874, 73.9453)
  point P3 (-25.3874, -40.0547)
  point P4 (-3.0874, 63.9453)
  point P5 (52.9126, 0.9453)
  point P6 (52.9126, 25.9453)
  point P7 (6.9126, 22.9453)
  point P8 (11.9126, 18.5453)
  point P9 (-25.3874, 73.9453)
  point P10 (-25.3874, 72.9453)
  point P11 (95.2126, 72.9453)
  point P12 (95.2126, 73.9453)
  point P13 (6.9126, -2.0547)
  point P14 (-25.5874, 62.9453)
  point P15 (85.4126, 62.9453)
  point P16 (6.9126, 10.6953)
  point P17 (25.6626, 63.9453)
  point P18 (34.1626, 63.9453)
  point P19 (25.6626, -40.0547)
  dimension "d704" = 1
  dimension "d707" = 1
  dimension "d710" = 0
  dimension "d711" = 1
  dimension "d712" = 0
  dimension "d713" = 0
  dimension "d719" = 0
  dimension "d720" = 0
  dimension "d721" = 1
  dimension "d722" = 0
  dimension "d787" = 2
  dimension "d788" = 1
  dimension "d789" = 2
  dimension "d790" = 1
  constraints: 48 end point, 12 parallel, 6 horizontal, 6 perpendicular, 1 point on line, 2 other
  measures "d704" distance between parallel lines of L0 L2
  measures "d707" distance between parallel lines of L7 L9
  measures "d710" distance between parallel lines of L20 L13
  measures "d711" distance between parallel lines of L13 L15
  measures "d712" distance between parallel lines of L21 L12
  measures "d713" distance between parallel lines of L22 L14
  measures "d719" distance between parallel lines of L23 L18
  measures "d720" horizontal extent of L17
  measures "d722" distance between parallel lines of L25 L16
  measures "d787" distance of L28.end L29.end
  measures "d788" distance of L27.end L28.end
  measures "d789" distance of L34.end L33.end
  measures "d790" distance of L33.end L32.end
extrude "Extrusion71" cut sketch "Sketch73" along normal blind 0.45 from surface at -1.4 contours L0 L31 L2 L3 | L0 L1 L2 L31 | L9 L6 L7 L4 | L12 L13 L14 L15 | L19 L18 L17 L16 | L28 L29 L30 L26 | L31 L34 L33 L32
chamfer "Chamfer30" distance 2.5 angle 45 1 edges at (22.1626, 11.9453, -8)
chamfer "Chamfer32" distance 0.7 angle 45 1 edges at (19.6376, 11.9453, 5)
sketch "Sketch76" plane through (0, 0, 5) normal (0, 0, 1) x (1, 0, 0)
  line L0 (89.9126, 71.9453) -> (88.4126, 71.9453)
  line L1 (88.4126, 71.9453) -> (88.4126, -48.0547)
  line L2 (88.4126, -48.0547) -> (89.9126, -48.0547)
  line L3 (89.9126, -48.0547) -> (89.9126, 71.9453)
  line L4 (89.9126, -48.0547) -> (89.9126, 71.9453) projected
  line L5 (89.9126, 71.9453) -> (-30.0874, 71.9453) projected
  line L6 (-30.0874, -48.0547) -> (89.9126, -48.0547) projected
  line L7 (-30.0874, 71.9453) -> (-28.5874, 71.9453)
  line L8 (-28.5874, 71.9453) -> (-28.5874, -48.0547)
  line L9 (-28.5874, -48.0547) -> (-30.0874, -48.0547)
  line L10 (-30.0874, -48.0547) -> (-30.0874, 71.9453)
  line L11 (-30.0874, 71.9453) -> (-30.0874, 63.9453) projected
  point P0 (0, 0)
  point P1 (89.9126, 63.9453)
  point P2 (-30.0874, 71.9453)
  dimension "d777" = 0
  dimension "d778" = 1.5
  dimension "d779" = 0
  dimension "d780" = 0
  dimension "d781" = 0
  dimension "d782" = 0
  dimension "d783" = 1.5
  dimension "d784" = 0
  constraints: 16 end point, 4 parallel, 2 horizontal, 2 perpendicular
  measures "d777" distance between parallel lines of L4 L3
  measures "d778" distance between parallel lines of L3 L1
  measures "d779" distance between parallel lines of L5 L0
  measures "d780" distance between parallel lines of L6 L2
  measures "d781" distance between parallel lines of L5 L7
  measures "d782" distance between parallel lines of L11 L10
  measures "d783" distance between parallel lines of L10 L8
  measures "d784" distance between parallel lines of L6 L9
extrude "Extrusion74" add sketch "Sketch76" against normal up to surface (7.5 mm away) contours L3 L2 L1 L0 | L8 L6 L10 L5
equation "\"d9\" = d15"
equation "\"d19\" = d56"
equation "\"d20\" = d56"
equation "\"d23\" = d56"
equation "\"d24\" = d32"
equation "\"d25\" = d32"
equation "\"d28\" = d33"
equation "\"d29\" = d33"
equation "\"d30\" = d33"
equation "\"d31\" = d32"
equation "\"d58\" = d15"
equation "\"d49\" = d51"
equation "\"d66\" = d62"
body "Solid1"
